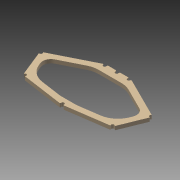
# Autodesk Inventor part: section1
Saved by Autodesk Inventor 2015 (Build 190159000, 159)
## iProperties
Created: 2017-09-23
Part Number: section1
Material: Polyethylene, High Density
Document SubType Name: Modeling
Designer: Mimoja
Density: 0.952 g/cm^3
Appearance: Smooth - Off-White
Mass: 636.712 g
Surface Area: 1195.02 cm^2
Volume: 668.815 cm^3
Author: Mimoja
Autodesk Inventor part; units mm, degrees
ref_plane "YZ Plane" through (0, 0, 0) normal (1, 0, 0) x (0, 1, 0)
ref_plane "XZ Plane" through (0, 0, 0) normal (0, 1, 0) x (-1, 0, 0)
ref_plane "XY Plane" through (0, 0, 0) normal (0, 0, 1) x (1, 0, 0)
sketch "Sketch1" plane through (0, 0, 0) normal (0, 0, 1) x (1, 0, 0)
  line L0 (0, 1.2192) -> (-219.456, 32.9184)
  line L1 (-219.456, 32.9184) -> (-275.5392, 172.212)
  line L2 (-275.5392, 172.212) -> (-60.96, 279.1968)
  line L3 (0, 569.8709) -> (0, -138.2601) construction
  line L4 (-60.96, 279.1968) -> (0, 279.1968)
  line L5 (0, 279.1968) -> (0, 1.2192)
  point P0 (0, 0)
  dimension "d9" = 279.1968
  dimension "d11" = 275.5392
  dimension "d15" = 172.212
  dimension "d20" = 219.456
  dimension "d22" = 32.9184
  dimension "d39" = 60.96
  dimension "d41" = 0
  dimension "d42" = 1.2192
  constraints: 12 end point, 1 collinear, 1 perpendicular, 1 point on line, 1 vertical
  measures "d9" vertical distance of point (0, 0) L2.end
  measures "d11" horizontal distance of point (0, 0) L1.end
  measures "d15" vertical distance of point (0, 0) L1.end
  measures "d20" horizontal distance of point (0, 0) L0.end
  measures "d22" vertical distance of point (0, 0) L0.end
  measures "d39" horizontal distance of point (0, 0) L2.end
  measures "d41" horizontal distance of point (0, 0) L0.start
  measures "d42" distance of point (0, 0) L0.start
extrude "Extrusion4" add sketch "Sketch1" along normal blind 18
hole "Hole2" at (0.0182, 271.8379, 18) direction (0, 0, -1) diameter 15 end through all
hole "Hole3" at (-269.2376, 170.2432, 18) direction (0, 0, -1) diameter 15 end through all
hole "Hole4" at (-214.5681, 37.3604, 18) direction (0, 0, -1) diameter 15 end through all
hole "Hole5" at (0.2097, 7.9943, 18) direction (0, 0, -1) diameter 15 end through all
hole "Hole6" at (-58.7896, 272.26, 18) direction (0, 0, -1) diameter 15 end through all
fillet "Fillet6" radius 5 1 edges at (-1.43, 279.1968, 9)
fillet "Fillet7" radius 3 1 edges at (-55.9383, 279.1968, 9)
fillet "Fillet8" radius 3 1 edges at (-63.9419, 277.7101, 9)
fillet "Fillet9" radius 1 1 edges at (-265.9589, 176.9885, 9)
fillet "Fillet10" radius 1 1 edges at (-271.9277, 163.2422, 9)
fillet "Fillet11" radius 1 1 edges at (-221.8931, 38.9713, 9)
fillet "Fillet12" radius 1 1 edges at (-209.8495, 31.5308, 9)
fillet "Fillet13" radius 3.5 1 edges at (-4.0184, 1.7996, 9)
sketch "Sketch4" plane through (0, 0, 18) normal (0, 0, 1) x (1, 0, 0)
  line L0 (-40, 35.2876) -> (-199.5017, 58.3267)
  line L1 (-199.5017, 58.3267) -> (-239.9101, 158.6888)
  line L2 (-239.9101, 158.6888) -> (-80, 238.4167)
  line L3 (-80, 238.4167) -> (0, 238.4167)
  line L4 (-40, 35.2876) -> (0, 35.2876)
  line L5 (0, 15.4913) -> (0, 264.338) projected
  line L6 (0, 238.4167) -> (0, 35.2876)
  line L7 (-70.6132, 274.3839) -> (-264.3764, 177.7775) projected
  line L8 (-271.1992, 161.4328) -> (-222.8264, 41.2894) projected
  line L9 (-207.9246, 31.2527) -> (-11.1586, 2.831) projected
  point P0 (0, 0)
  dimension "d171" = 28
  dimension "d172" = 28
  dimension "d173" = 28
  dimension "d174" = 40
  dimension "d175" = 80
  constraints: 12 end point, 3 parallel, 2 horizontal, 1 perpendicular, 1 point on line
  measures "d171" distance between parallel lines of L7 L2
  measures "d172" distance between parallel lines of L8 L1
  measures "d173" distance between parallel lines of L9 L0
  measures "d174" distance of L0.start L4.end
  measures "d175" distance of L2.end L3.end
extrude "Extrusion5" cut sketch "Sketch4" against normal through all
fillet "Fillet14" radius 40 1 edges at (-239.9101, 158.6888, 9)
fillet "Fillet15" radius 100 1 edges at (-80, 238.4167, 9)
fillet "Fillet16" radius 100 1 edges at (-199.5017, 58.3267, 9)
fillet "Fillet17" radius 100 1 edges at (-40, 35.2876, 9)
mirror "Mirror3" about plane through (0, 0, 0) normal (1, 0, 0)
body "Solid4"
